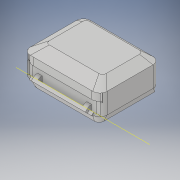
# Autodesk Inventor part: printer
Saved by Autodesk Inventor 2017 (Build 210142000, 142)
## iProperties
Created: 2018-04-03
Part Number: printer
Material: Generic
Document SubType Name: Modeling
Designer: Braxton
Density: 1 g/cm^3
Appearance: Default
Author: Braxton
Autodesk Inventor part; units mm, degrees
ref_plane "XZ Plane" through (0, 0, 0) normal (0, 1, 0) x (-1, 0, 0)
ref_plane "XY Plane" through (0, 0, 0) normal (0, 0, 1) x (1, 0, 0)
sketch "Sketch1" plane through (0, 0, 0) normal (0, 1, 0) x (-1, 0, 0)
  line L0 (20.6375, 12.3693) -> (20.6375, -12.3693)
  line L1 (16.801, 16.2057) -> (0, 16.2057)
  line L2 (0, 0) -> (0, 16.2057) construction
  line L3 (16.801, -16.2057) -> (0, -16.2057)
  arc A0 (16.801, -16.2057) -> (20.6375, -12.3693) centre (16.801, -12.3693) ccw
  arc A1 (20.6375, 12.3693) -> (16.801, 16.2057) centre (16.801, 12.3693) ccw
  line L4 (20.6375, 0) -> (0, 0) construction
  line L5 (-20.6375, 12.3693) -> (-20.6375, -12.3693)
  line L6 (-16.801, 16.2057) -> (0, 16.2057)
  line L7 (-16.801, -16.2057) -> (0, -16.2057)
  arc A2 (-20.6375, -12.3693) -> (-16.801, -16.2057) centre (-16.801, -12.3693) ccw
  arc A3 (-16.801, 16.2057) -> (-20.6375, 12.3693) centre (-16.801, 12.3693) ccw
  line L8 (-20.6375, 0) -> (0, 0) construction
  dimension "d3" = 3.8365
  dimension "d4" = 32.4115
  dimension "d5" = 3.8365
  dimension "d6" = 20.6375
  constraints: 18 end point, 8 point on circle, 7 symmetric about line, 4 centre point, 4 tangent, 3 perpendicular, 1 coincident, 1 horizontal, 1 midpoint, 1 point on line, 2 other
  measures "d3" radius of A0
  measures "d4" distance between parallel lines of L1 L3
  measures "d5" radius of A1
  measures "d6" distance from line of L1.end L0
extrude "middle of body" add sketch "Sketch1" along normal blind 11.0384
ref_plane "top of printer" through (0, 14.2304, 0) normal (0, 1, 0) x (1, 0, 0)
sketch "Sketch2" plane through (0, 14.2304, 0) normal (0, 1, 0) x (1, 0, 0)
  line L0 (-13.3615, -9.4589) -> (0, -9.4589)
  line L1 (0, 12.3693) -> (-13.3615, 12.3693)
  line L2 (-15.2797, 10.451) -> (-15.2797, -7.5406)
  arc A0 (-15.2797, -7.5406) -> (-13.3615, -9.4589) centre (-13.3615, -7.5406) ccw
  arc A1 (-13.3615, 12.3693) -> (-15.2797, 10.451) centre (-13.3615, 10.451) ccw
  line L3 (0, -9.4589) -> (0, 0) construction
  line L4 (0, 0) -> (0, 12.3693) construction
  line L5 (16.801, 16.2057) -> (-16.801, 16.2057) projected
  line L6 (13.3615, -9.4589) -> (0, -9.4589)
  line L7 (0, 12.3693) -> (13.3615, 12.3693)
  line L8 (15.2797, 10.451) -> (15.2797, -7.5406)
  arc A2 (13.3615, -9.4589) -> (15.2797, -7.5406) centre (13.3615, -7.5406) ccw
  arc A3 (15.2797, 10.451) -> (13.3615, 12.3693) centre (13.3615, 10.451) ccw
  dimension "d10" = 15.2797
  dimension "d11" = 21.8281
  dimension "d12" = 3.8365
  dimension "d13" = 1.9182
  constraints: 16 end point, 8 point on circle, 6 symmetric about line, 4 centre point, 4 tangent, 2 perpendicular, 1 coincident, 1 collinear, 1 equal radius, 2 other
  measures "d10" distance from line of L1.start L2
  measures "d11" distance between parallel lines of L0 L1
  measures "d12" distance between parallel lines of L5 L1
  measures "d13" radius of A1
loft "top part of printer" add profiles "Sketch2" section 1 edges at (8.4005, 11.0384, 16.2057) (-8.4005, 11.0384, 16.2057) (19.5138, 11.0384, 15.0821) (20.6375, 11.0384, 0) (19.5138, 11.0384, -15.0821) (-8.4005, 11.0384, -16.2057) (8.4005, 11.0384, -16.2057) (-19.5138, 11.0384, -15.0821) (-20.6375, 11.0384, 0) (-19.5138, 11.0384, 15.0821)
ref_plane "Bottom of printer" through (0, -4.5328, 0) normal (0, -1, 0) x (1, 0, 0)
sketch "Sketch3" plane through (0, -4.5328, 0) normal (0, -1, 0) x (1, 0, 0)
  line L0 (16.801, -16.2057) -> (-16.801, -16.2057) projected
  line L1 (-18.124, -15.9704) -> (-18.124, 11.5314)
  line L2 (-15.5663, 14.0891) -> (0, 14.0891)
  line L3 (0, 14.0891) -> (0, -16.2057) construction
  arc A0 (-15.5663, 14.0891) -> (-18.124, 11.5314) centre (-15.5663, 11.5314) ccw
  line L4 (-16.801, 16.2057) -> (16.801, 16.2057) projected
  line L5 (-16.801, -16.2057) -> (0, -16.2057)
  line L6 (18.124, -15.9704) -> (18.124, 11.5314)
  line L7 (15.5663, 14.0891) -> (0, 14.0891)
  arc A1 (18.124, 11.5314) -> (15.5663, 14.0891) centre (15.5663, 11.5314) ccw
  line L8 (16.801, -16.2057) -> (0, -16.2057)
  line L9 (16.801, -16.2057) -> (-16.801, -16.2057) projected
  arc A2 (16.801, -16.2057) -> (20.6375, -12.3693) centre (16.801, -12.3693) ccw projected
  arc A3 (16.801, -16.2057) -> (18.124, -15.9704) centre (16.801, -12.3693) ccw
  arc A4 (-20.6375, -12.3693) -> (-16.801, -16.2057) centre (-16.801, -12.3693) ccw projected
  arc A5 (-18.124, -15.9704) -> (-16.801, -16.2057) centre (-16.801, -12.3693) ccw
  point P0 (0, 0)
  dimension "d19" = 18.124
  dimension "d21" = 2.1167
  dimension "d22" = 2.5576
  constraints: 14 end point, 12 point on circle, 4 centre point, 3 symmetric about line, 3 tangent, 3 vertical, 2 concentric, 1 midpoint, 1 perpendicular, 1 other
  measures "d19" distance from line of L2.end L1
  measures "d21" distance between parallel lines of L4 L2
  measures "d22" radius of A0
loft "bottom part of printer" add profiles "Sketch3" section 1 edges at (0, 0, 16.2057) (-19.5138, 0, 15.0821) (-20.6375, 0, 0) (-19.5138, 0, -15.0821) (0, 0, -16.2057) (19.5138, 0, -15.0821) (20.6375, 0, 0) (19.5138, 0, 15.0821)
sketch "Sketch7" plane through (0, 0, 0) normal (0, 1, 0) x (-1, 0, 0)
  line L0 (17.2445, 14.6352) -> (0, 14.6352)
  arc A0 (18.9061, 14.3929) -> (17.2445, 14.6352) centre (17.2445, 8.8168) ccw
  line L1 (0, 14.6352) -> (0, 0) construction
  line L2 (16.801, 16.2057) -> (-16.801, 16.2057) projected
  line L3 (20.6375, -12.3693) -> (20.6375, 12.3693) projected
  line L4 (18.9061, 14.3929) -> (19.5668, 15.028)
  arc A1 (20.6375, 12.3693) -> (16.801, 16.2057) centre (16.801, 12.3693) ccw projected
  arc A2 (19.5668, 15.028) -> (16.801, 16.2057) centre (16.801, 12.3693) ccw
  line L5 (16.801, 16.2057) -> (13.3615, 9.4589) projected
  line L6 (16.801, 16.2057) -> (0, 16.2057)
  line L7 (-17.2445, 14.6352) -> (0, 14.6352)
  arc A3 (-17.2445, 14.6352) -> (-18.9061, 14.3929) centre (-17.2445, 8.8168) ccw
  line L8 (-18.9061, 14.3929) -> (-19.5668, 15.028)
  arc A4 (-16.801, 16.2057) -> (-19.5668, 15.028) centre (-16.801, 12.3693) ccw
  line L9 (-16.801, 16.2057) -> (0, 16.2057)
  point P0 (-16.801, 12.3693)
  dimension "d43" = 1.5706
  dimension "d46" = 0.4434
  dimension "d47" = 0.9165
  dimension "d48" = 1.7314
  dimension "d87" = 33.6021
  constraints: 14 end point, 9 point on circle, 6 symmetric about line, 4 centre point, 1 concentric, 1 horizontal, 1 line through centre, 1 midpoint, 1 tangent, 1 vertical, 2 other
  measures "d43" distance between parallel lines of L2 L0
  measures "d46" horizontal distance of L0.start L2.start
  measures "d47" distance of L4.start L4.end
  measures "d48" distance from line of L3 L4.start
  measures "d87" distance of L2.end L2.start
extrude "front bottom door slot" cut sketch "Sketch7" along normal blind 6.4537
sketch "Sketch9" plane through (0, 6.4537, 0) normal (0, -1, 0) x (1, 0, 0)
  line L0 (-16.801, 16.2057) -> (16.801, 16.2057) projected
  line L1 (0, 16.2057) -> (-16.801, 16.2057)
  arc A0 (-19.5668, 15.028) -> (-20.6375, 12.3693) centre (-16.801, 12.3693) ccw projected
  arc A1 (-16.801, 16.2057) -> (-20.1955, 14.1569) centre (-16.801, 12.3693) ccw
  line L2 (0, 15.7443) -> (-15.5183, 15.7443)
  line L3 (0, 16.2057) -> (0, 15.7443) construction
  line L4 (17.2445, 14.6352) -> (-17.2445, 14.6352) projected
  line L5 (-20.6375, -12.3693) -> (-20.6375, 12.3693) projected
  line L6 (-20.1955, 14.1569) -> (-19.8772, 13.9893)
  arc A2 (-15.5183, 15.7443) -> (-18.9061, 14.3929) centre (-15.5183, 10.8225) ccw
  line L7 (-18.9061, 14.3929) -> (-19.8772, 13.9893)
  line L8 (0, 16.2057) -> (16.801, 16.2057)
  arc A3 (20.1955, 14.1569) -> (16.801, 16.2057) centre (16.801, 12.3693) ccw
  line L9 (0, 15.7443) -> (15.5183, 15.7443)
  line L10 (20.1955, 14.1569) -> (19.8772, 13.9893)
  arc A4 (18.9061, 14.3929) -> (15.5183, 15.7443) centre (15.5183, 10.8225) ccw
  line L11 (18.9061, 14.3929) -> (19.8772, 13.9893)
  point P0 (0, 0)
  point P1 (19.5668, 15.028)
  point P2 (16.801, 12.3693)
  dimension "d57" = 1.1091
  dimension "d62" = 0.3598
  dimension "d63" = 1.8415
  dimension "d64" = 1.2827
  constraints: 18 end point, 9 point on circle, 8 symmetric about line, 4 centre point, 1 collinear, 1 concentric, 1 horizontal, 1 line through centre, 1 midpoint, 1 perpendicular, 1 tangent, 2 other
  measures "d57" distance between parallel lines of L4 L2
  measures "d62" distance of L6.start L6.end
  measures "d63" distance of L6.start L5.end
  measures "d64" horizontal distance of L2.end L0.start
extrude "front top door slot" cut sketch "Sketch9" against normal blind 4.5847
sketch "Sketch4" plane through (16.801, 11.0384, -16.2057) normal (0, 0, -1) x (-1, 0, 0)
  line L0 (37.4385, -15.5713) -> (37.4385, -5.8028)
  line L1 (37.4385, -11.0384) -> (37.4385, 0) projected
  line L2 (37.4385, -5.8028) -> (34.0117, -5.8028)
  line L3 (33.6137, -6.2008) -> (33.6137, -7.3745)
  line L4 (33.6021, -15.5713) -> (0, -15.5713) projected
  line L5 (37.4385, -15.5713) -> (28.0617, -15.5713)
  line L6 (28.0617, -15.5713) -> (28.0617, -9.4435)
  line L7 (29.5857, -7.9195) -> (33.0687, -7.9195)
  arc A0 (29.5857, -7.9195) -> (28.0617, -9.4435) centre (29.5857, -9.4435) ccw
  arc A1 (33.0687, -7.9195) -> (33.6137, -7.3745) centre (33.0687, -7.3745) ccw
  arc A2 (34.0117, -5.8028) -> (33.6137, -6.2008) centre (34.0117, -6.2008) ccw
  point P0 (16.801, -11.0384)
  dimension "d27" = 9.7684
  dimension "d30" = 9.3768
  dimension "d33" = 2.1167
  dimension "d36" = 1.524
  dimension "d37" = 0.545
  dimension "d38" = 0.3979
  dimension "d39" = 3.8248
  constraints: 12 end point, 6 point on circle, 6 tangent, 3 centre point, 3 vertical, 2 point on line, 1 collinear, 1 horizontal, 1 perpendicular
  measures "d27" distance of L0.start L0.end
  measures "d30" distance of L0.start L5.end
  measures "d33" distance between parallel lines of L2 L7
  measures "d36" radius of A0
  measures "d37" radius of A1
  measures "d38" radius of A2
  measures "d39" distance between parallel lines of L0 L3
extrude "cords cut" cut sketch "Sketch4" against normal blind 2.9401
sketch "Sketch5" plane through (-16.8127, 3.664, -16.2057) normal (-1, 0, 0) x (0, 0, 1)
  arc A0 (2.94, 0.3503) -> (1.7187, 1.5716) centre (1.7187, 0.3503) ccw
  line L0 (2.94, 1.5716) -> (0.0219, 1.5716) projected
  line L1 (2.94, 1.5716) -> (0, 1.5716)
  line L2 (2.94, 0.3503) -> (2.94, 1.5716)
  line L3 (2.94, 1.5716) -> (1.7187, 1.5716)
  point P0 (16.2057, -3.664)
  dimension "d40" = 1.2213
  constraints: 6 end point, 2 point on circle, 2 tangent, 1 centre point, 1 horizontal, 1 perpendicular, 1 vertical
  measures "d40" radius of A0
extrude "cords join curve part" add sketch "Sketch5" along normal up to surface round surface about axis through (-16.801, 0, -12.3693) along (0, 1, 0) radius 3.8365 far side no
ref_plane "rack rotation Work Plane" through (12.0385, 0, 0) normal (1, 0, 0) x (0, 1, 0)
sketch "Sketch10" plane through (12.0385, 0, 0) normal (1, 0, 0) x (0, 1, 0)
  line L0 (0, 15.028) -> (6.4537, 15.028) projected
  line L1 (0, 14.6352) -> (6.4537, 14.6352) projected
  line L2 (2.168, 16.8031) -> (0, 14.6352)
  line L3 (0, 14.6352) -> (3.066, 14.6352)
  arc A0 (3.066, 14.6352) -> (2.168, 16.8031) centre (0, 14.6352) ccw
  point P0 (0, 0)
  point P1 (0, 16.2057)
  dimension "d72" = 3.066
  dimension "d74" = 45
  constraints: 4 end point, 2 point on circle, 1 centre point, 1 coincident, 1 horizontal
  measures "d72" radius of A0
  measures "d74" angle of L3 L2
extrude "rack rotation" add sketch "Sketch10" along normal blind 2.5019
mirror "Mirror of rack rotation" about plane through (0, 0, 0) normal (1, 0, 0) of "rack rotation"
sketch "Sketch11" plane through (12.0385, 1.0046, 15.6398) normal (0, -0.7071068, 0.7071068) x (1, 0, 0)
  line L0 (3.4798, 7.1688) -> (-27.5569, 7.1688) projected
  line L1 (-26.579, 1.6452) -> (2.5019, 1.6452)
  line L2 (-26.579, 0.7472) -> (-26.579, 1.6452) projected
  line L3 (-26.579, 1.6452) -> (-26.579, 0.1498)
  line L4 (-26.579, 0.1498) -> (2.5019, 0.1498)
  line L5 (2.5019, 1.6452) -> (2.5019, 0.1498)
  line L6 (2.5019, 0.7472) -> (2.5019, 1.6452) projected
  point P0 (-12.0385, -11.7694)
  dimension "d95" = 1.4954
  constraints: 8 end point, 1 collinear, 1 point on line
  measures "d95" distance of L1.end L4.end
extrude "connection to rack rotations" add sketch "Sketch11" along normal blind 1.5706
ref_plane "tray work plane" through (12.0385, 2.168, 16.8031) normal (0, -0.7071068, 0.7071068) x (1, 0, 0)
sketch "Sketch14" plane through (0, 0, 0) normal (1, 0, 0) x (0, 1, 0)
  line L0 (0, 16.8563) -> (1.0574, 17.9137) projected
  line L1 (1.1106, 15.7457) -> (0, 16.8563)
  line L2 (1.1106, 15.7457) -> (0, 16.8563)
  line L3 (1.1106, 15.7457) -> (-0.5186, 16.3377)
  line L4 (0, 16.8563) -> (-0.5186, 16.3377)
  point P0 (0, 0)
  dimension "d93" = 0.7334
  dimension "d94" = 1.5706
  constraints: 8 end point, 2 collinear, 1 perpendicular
  measures "d93" distance of L0.start L3.end
  measures "d94" distance of L0.start L1.start
extrude "rest for tray" add sketch "Sketch14" along normal mid plane 33.6021
equation "\"d5\" = d3"
equation "\"d13\" = 0.5 * d3"
equation "\"d22\" = 0.666667 * d3"
body "Solid1"
